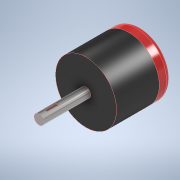
# Autodesk Inventor part: Rotator_N5065
Saved by Autodesk Inventor 2021 (Build 250183000, 183)
## iProperties
Created: 2020-08-28
Part Number: Rotator_N5065
Material: Generic
Document SubType Name: Modeling
Designer: Hagihara Yuya
Density: 1 g/cm^3
Appearance: 赤
Author: Hagihara Yuya
Autodesk Inventor part; units mm, degrees
ref_plane "YZ Plane" through (0, 0, 0) normal (1, 0, 0) x (0, 1, 0)
sketch "スケッチ1" plane through (0, 0, 0) normal (0, 0, 1) x (1, 0, 0)
  circle A0 centre (0, 0) radius 25
  dimension "d0" = 50
  constraints: 1 centre point, 1 coincident
  measures "d0" diameter of A0
extrude "押し出し1" add sketch "スケッチ1" against normal blind 10
fillet "フィレット1" radius 4 1 edges at (-25, 0, -10)
sketch "スケッチ2" plane through (0, 0, 0) normal (0, 0, 1) x (1, 0, 0)
  circle A0 centre (0, 0) radius 25
  circle A1 centre (0, 0) radius 25 projected
  constraints: 1 centre point, 1 coincident, 1 concentric
extrude "押し出し2" add sketch "スケッチ2" along normal blind 35
sketch "スケッチ3" plane through (0, 0, 0) normal (0, 0, 1) x (1, 0, 0)
  circle A0 centre (0, 0) radius 25
  circle A1 centre (0, 0) radius 25 projected
  circle A2 centre (0, 0) radius 24.99
  dimension "d6" = 0.01
  constraints: 2 centre point, 2 coincident, 1 concentric
  measures "d6" radial gap between concentric circles of A0 A2
extrude "押し出し3" cut sketch "スケッチ3" against normal blind 0.01
sketch "スケッチ4" plane through (0, 0, -10) normal (0, 0, -1) x (-1, 0, 0)
  point P0 (0, 0)
  point P1 (0, 0)
  constraints: 1 coincident
hole "穴1" at (0, 0, -10) direction (0, 0, 1) diameter 8 end through all
sketch "スケッチ5" plane through (0, 0, -10) normal (0, 0, -1) x (-1, 0, 0)
  point P0 (0, 0)
  point P1 (0, -10)
  point P2 (10, 0)
  point P3 (0, 10)
  point P4 (-10, 0)
  dimension "d18" = 360
  dimension "d20" = 20
  constraints: 1 vertical alignment, 5 other
  measures "d20" distance of point (0, 10) point (0, -10)
hole "穴2" at (0, -10, -10) at (-10, 0, -10) at (0, 10, -10) at (10, 0, -10) direction (0, 0, 1) diameter 3.242 depth 11.8 tip angle 118 thread size "M4x0.7" class "6H" standard "ISO Metric profile"
ref_plane "作業平面1" through (0, 0, -5) normal (0, 0, -1) x (-1, 0, 0)
sketch "スケッチ6" plane through (0, 0, -5) normal (0, 0, -1) x (-1, 0, 0)
  circle A0 centre (0, 0) radius 4 projected
  circle A1 centre (0, 0) radius 4
  dimension "d29" = 8
  constraints: 1 centre point, 1 coincident
  measures "d29" diameter of A1
extrude "押し出し4" add sketch "スケッチ6" against normal blind 78.5
ref_plane "作業平面2" through (0, 0, 68.5) normal (0, 0, 1) x (1, 0, 0)
sketch "スケッチ7" plane through (0, 0, 68.5) normal (0, 0, 1) x (1, 0, 0)
  line L0 (-1.5, 4) -> (1.5, 4)
  line L1 (1.5, 4) -> (1.5, 2.5)
  line L2 (1.5, 2.5) -> (-1.5, 2.5)
  line L3 (-1.5, 2.5) -> (-1.5, 4)
  circle A0 centre (0, 0) radius 4 projected
  point P0 (0, 2.5)
  dimension "d33" = 3
  dimension "d34" = 1.5
  constraints: 8 end point, 2 parallel, 1 horizontal, 1 midpoint, 1 perpendicular, 1 tangent, 1 vertical alignment
  measures "d33" distance of L0.start L0.end
  measures "d34" distance of L0.end L1.end
extrude "押し出し5" cut sketch "スケッチ7" against normal blind 10 contours L0 A0 L3 | L0 L1 A0 | A0 L1 L2 L3 picked at (0, 3)
